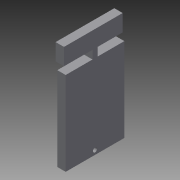
# Autodesk Inventor part: Stresstest
Saved by Autodesk Inventor 2015 (Build 190159000, 159)
## iProperties
Created: 2017-01-06
Part Number: Stresstest
Material: Generic
Document SubType Name: Modeling
Designer: Rudge-Top
Density: 1 g/cm^3
Appearance: Default
Author: Rudge-Top
Autodesk Inventor part; units mm, degrees
ref_plane "YZ Plane" through (0, 0, 0) normal (1, 0, 0) x (0, 1, 0)
ref_plane "XZ Plane" through (0, 0, 0) normal (0, 1, 0) x (-1, 0, 0)
ref_plane "XY Plane" through (0, 0, 0) normal (0, 0, 1) x (1, 0, 0)
sketch "Sketch1" plane through (0, 0, 0) normal (1, 0, 0) x (0, 1, 0)
  line L0 (0, 0) -> (35, 0)
  line L1 (35, 0) -> (35, -50)
  line L2 (35, -50) -> (0, -50)
  line L3 (0, -50) -> (0, 0)
  line L4 (17.5, 0) -> (17.5, 11.9434)
  line L5 (19, 0) -> (19, 5)
  line L6 (16, 0) -> (16, 5)
  line L7 (-1, 5) -> (34, 5)
  line L8 (34, 5) -> (34, 15)
  line L9 (34, 15) -> (-1, 15)
  line L10 (-1, 15) -> (-1, 5)
  line L11 (16, 5) -> (19, 5)
  line L12 (19, 0) -> (16, 0)
  dimension "d0" = 35
  dimension "d1" = 50
  dimension "d2" = 5
  dimension "d3" = 1.5
  dimension "d4" = 1.5
  dimension "d11" = 10
  dimension "d12" = 0
  constraints: 26 end point, 6 parallel, 2 horizontal, 2 perpendicular, 2 point on line, 2 vertical, 1 collinear, 1 midpoint
  measures "d0" distance of L1.end L2.end
  measures "d1" distance of L2.end L0.start
  measures "d2" distance of L5.start L5.end
  measures "d3" distance between parallel lines of L4 L6
  measures "d4" distance between parallel lines of L5 L4
  measures "d11" distance of L7.end L8.end
  measures "d12" distance from line of L5.end L7
extrude "Extrusion1" add sketch "Sketch1" along normal blind 5
sketch "Sketch3" plane through (5, 0, 0) normal (1, 0, 0) x (0, 0, -1)
  circle A0 centre (47.5, 17.5) radius 1.25
  line L0 (50, 0) -> (50, 35) projected
  line L1 (0, 0) -> (50, 0) projected
  dimension "d16" = 2.5
  dimension "d17" = 2.5
  dimension "d18" = 17.5
  constraints: 1 centre point
  measures "d16" diameter of A0
  measures "d17" distance from line of L0 A0.centre
  measures "d18" distance from line of L1 A0.centre
extrude "Extrusion3" cut sketch "Sketch3" against normal blind 5
equation "\"d3\" = 0.5 * Snap"
equation "\"d4\" = 0.5 * Snap"
equation "\"Snap\" = 3"
body "Solid1"
